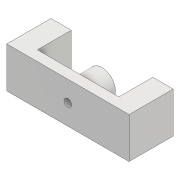
# Autodesk Inventor part: Support_Holder
Saved by Autodesk Inventor 2017 (Build 210142000, 142)
## iProperties
Created: 2017-07-03
Part Number: Support_Holder
Material: ABS Plastic
Document SubType Name: Modeling
Designer: Fran Rower
Mass: 2.3673 g
Surface Area: 19.8115 cm^2
Volume: 2.2333 cm^3
Density: 1.06 g/cm^3
Appearance: Smooth - White
Author: Fran Rower
Autodesk Inventor part; units mm, degrees
ref_plane "YZ Plane" through (0, 0, 0) normal (1, 0, 0) x (0, 1, 0)
ref_plane "XZ Plane" through (0, 0, 0) normal (0, 1, 0) x (-1, 0, 0)
ref_plane "XY Plane" through (0, 0, 0) normal (0, 0, 1) x (1, 0, 0)
sketch "Sketch1" plane through (0, 0, 0) normal (0, 0, 1) x (1, 0, 0)
  line L0 (0, 0) -> (18, 0)
  line L1 (18, 0) -> (18, 13)
  line L2 (18, 13) -> (12, 13)
  line L3 (12, 13) -> (12, 3)
  line L4 (12, 3) -> (0, 3)
  line L5 (0, 3) -> (0, 0) construction
  line L6 (0, 0) -> (-18, 0)
  line L7 (-18, 0) -> (-18, 13)
  line L8 (-18, 13) -> (-12, 13)
  line L9 (-12, 13) -> (-12, 3)
  line L10 (-12, 3) -> (0, 3)
  point P0 (15, 13)
  dimension "d2" = 6
  dimension "d3" = 3
  dimension "d4" = 13
  dimension "d18" = 15
  constraints: 22 end point, 4 perpendicular, 4 symmetric about line, 1 horizontal, 1 midpoint, 1 vertical
  measures "d2" distance of L1.end L2.end
  measures "d3" distance between parallel lines of L0 L4
  measures "d4" distance of L0.end L1.end
  measures "d18" horizontal distance of L0.start point (15, 13)
extrude "Extrusion1" add sketch "Sketch1" along normal blind 12
sketch "Sketch2" plane through (-18, 0, 0) normal (0, -1, 0) x (1, 0, 0)
  circle A0 centre (18, 6) radius 1.1
  line L0 (0, 0) -> (36, 0) projected
  line L1 (0, 0) -> (0, 12) projected
  point P0 (18, 0)
  dimension "d7" = 2.2
  dimension "d19" = 6
  dimension "d20" = 18
  constraints: 1 centre point
  measures "d7" diameter of A0
  measures "d19" distance from line of L0 A0.centre
  measures "d20" distance from line of L1 A0.centre
extrude "Extrusion2" cut sketch "Sketch2" against normal blind 12
sketch "Sketch3" plane through (-12, 3, 0) normal (0, 1, 0) x (1, 0, 0)
  circle A0 centre (12, -6) radius 1.1 projected
  circle A1 centre (12, -6) radius 4
  point P0 (12, 0)
  dimension "d11" = 8
  constraints: 1 centre point, 1 coincident
  measures "d11" diameter of A1
extrude "Extrusion3" add sketch "Sketch3" along normal blind 7
sketch "Sketch5" plane through (0, 0, 0) normal (0, 0, -1) x (-1, 0, 0)
  circle A0 centre (0, 6.6873) radius 1.1
  line L0 (-12, 3) -> (12, 3) projected
  point P0 (0, 3)
  dimension "d29" = 2.2
  constraints: 1 centre point, 1 midpoint, 1 vertical alignment
  measures "d29" diameter of A0
extrude "Extrusion5" cut sketch "Sketch5" against normal blind 5.75
equation "\"d19\" = 0.5 * d5"
equation "\"d20\" = d18 + 0.5 * d2"
equation "\"d5\" = 12"
body "Solid1"
